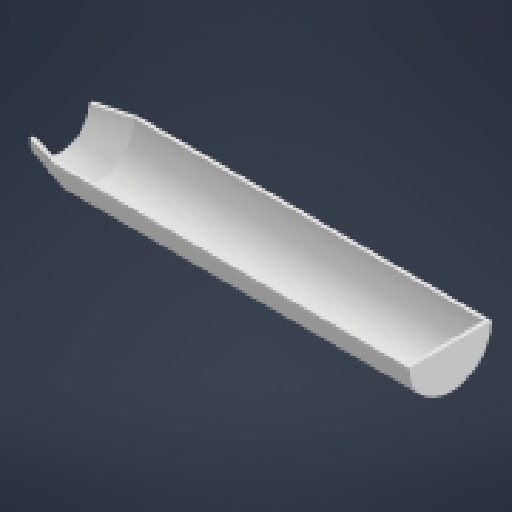
# Autodesk Inventor part: Half bottom
Saved by Autodesk Inventor 2023 (Build 270158000, 158)
## iProperties
Created: 2023-12-06
Part Number: Half bottom
Material: Generic
Document SubType Name: Modeling
Designer: Andi
Density: 1 g/cm^3
Appearance: Default
Author: Andi
Autodesk Inventor part; units mm, degrees
ref_plane "YZ Plane" through (0, 0, 0) normal (1, 0, 0) x (0, 1, 0)
ref_plane "XZ Plane" through (0, 0, 0) normal (0, 1, 0) x (-1, 0, 0)
ref_plane "XY Plane" through (0, 0, 0) normal (0, 0, 1) x (1, 0, 0)
sketch "Sketch1" plane through (0, 0, 0) normal (0, 1, 0) x (-1, 0, 0)
  line L0 (90, -21.0403) -> (-90, -21.0403)
  line L1 (-90, -21.0403) -> (-90, 0)
  line L2 (-90, 18.9597) -> (90, 18.9597) construction
  line L3 (90, -21.0403) -> (107.4444, -16.0403)
  line L4 (163.4072, 0) -> (107.4444, 13.9597) construction
  line L5 (107.4444, -16.0403) -> (107.4444, -13.9597)
  line L6 (107.4444, -16.0403) -> (163.4072, 0) construction
  line L7 (107.4444, 13.9597) -> (90, 18.9597) construction
  line L8 (163.4072, 0) -> (-90, 0)
  line L9 (-88, -19.0403) -> (89.719, -19.0403)
  line L10 (89.719, -19.0403) -> (107.4444, -13.9597)
  line L11 (-90, 0) -> (-88, 0)
  line L12 (-88, 0) -> (-88, -19.0403)
  line L13 (107.4444, 0) -> (107.4444, 13.9597) construction
  line L14 (-90, 0) -> (-90, 18.9597) construction
  line L15 (107.4444, -13.9597) -> (107.4444, 0) construction
  point P0 (0, 0)
  point P1 (108.6603, 0)
  dimension "d0" = 180
  dimension "d1" = 40
  dimension "d2" = 2
  dimension "d3" = 2
  dimension "d5" = 30
  dimension "d6" = 90
  dimension "d7" = 30
  dimension "d9" = 2
  constraints: 32 end point, 5 perpendicular, 3 equal length, 3 horizontal alignment, 3 vertical, 1 collinear, 1 horizontal, 1 parallel
  measures "d0" distance of L2.start L2.end
  measures "d1" distance of L0.end L2.start
  measures "d2" distance between parallel lines of L9 L0
  measures "d3" distance between parallel lines of L12 L1
  measures "d5" angle of L4 L6
  measures "d6" distance from line of point (0, 0) L1
  measures "d7" distance of L4.end L3.end
  measures "d9" distance between parallel lines of L10 L3
revolve "Revolution1" add sketch "Sketch1" angle 180 about axis through (-163.4072, 0, 0) along (-1, 0, 0)
equation "\"d3\" = d2"
equation "\"d9\" = d2"
body "Solid1"
